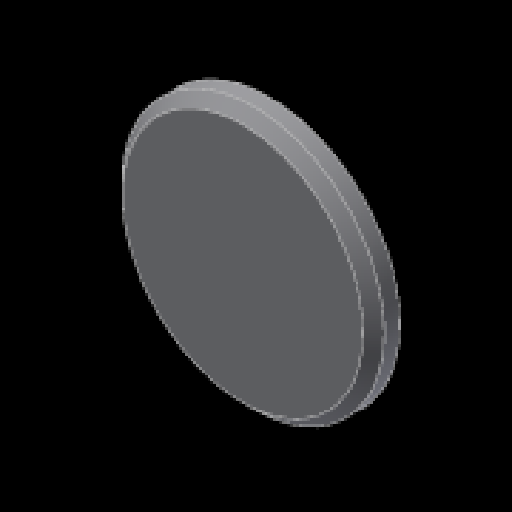
# Autodesk Inventor part: WheelEncoderCover
Saved by Autodesk Inventor 2025.2 (Build 292293000, 293)
## iProperties
Created: 2026-02-04
Part Number: WheelEncoderCover
Material: Generic
Document SubType Name: Modeling
Designer: valer
Density: 1 g/cm^3
Appearance: Default
Author: valer
Autodesk Inventor part; units mm, degrees
ref_plane "YZ Plane" through (0, 0, 0) normal (1, 0, 0) x (0, 1, 0)
ref_plane "XZ Plane" through (0, 0, 0) normal (0, 1, 0) x (-1, 0, 0)
ref_plane "XY Plane" through (0, 0, 0) normal (0, 0, 1) x (1, 0, 0)
sketch "Base" plane through (0, 0, 0) normal (0, 0, 1) x (1, 0, 0)
  circle A0 centre (0, 0) radius 21.75
  circle A1 centre (0, 0) radius 18.75
  circle A2 centre (0, 0) radius 20.25 construction
  dimension "d1" = 37.5
  dimension "d2" = 3
  dimension "d3" = 1.5
  constraints: 3 centre point, 3 coincident
  measures "d1" diameter of A1
  measures "d2" radial gap between concentric circles of A0 A1
  measures "d3" radial gap between concentric circles of A0 A2
extrude "BaseFeature" add sketch "Base" along normal blind 3
sketch "Cap" plane through (0, 0, 3) normal (0, 0, 1) x (1, 0, 0)
  circle A0 centre (0, 0) radius 21.75 projected
extrude "CapFeature" add sketch "Cap" along normal blind 2
chamfer "CapChamferFeature" distance 2 angle 45 1 edges at (-21.75, 0, 5)
sketch "MountHoles" plane through (0, 0, 5) normal (0, 0, 1) x (1, 0, 0)
  circle A0 centre (-4.0033, -15.0141) radius 1.25 projected
  circle A1 centre (15.0232, -3.9691) radius 1.25 projected
  circle A2 centre (4.0033, 15.0141) radius 1.25 projected
  circle A3 centre (-15.0232, 3.9691) radius 1.25 projected
  point P0 (0, 0)
extrude "MountHolesFeature" cut sketch "MountHoles" against normal blind 2
equation "\"d3\" = 0.5 * d2"
body "Solid1"
